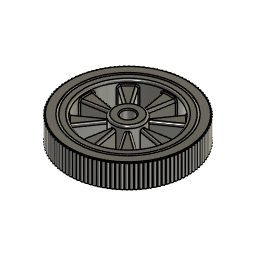
Reifen_Grip_V7 (Autodesk Fusion 360 design; units mm, degrees)
part number: 2025-05-07-17-34-55-146
Autodesk Fusion 360 part; units mm, degrees
note: some values were not read from the file. Chosen so that the rebuilt part matches the saved one: that a step has no effect.
sketch "Skizze1" plane through (0, 0, 0) normal (0, 0, 1) x (1, 0, 0)
  circle A0 centre (0, 0) radius 17
  circle A1 centre (0, 0) radius 14
  circle A2 centre (0, 0) radius 5
  circle A3 centre (0, 0) radius 2.1
  line L0 (-13.8696, -1.9063) -> (-7.5114, -0.5773)
  line L1 (16.2005, -5.1522) -> (10.483, -4.0435)
  line L2 (10.483, -4.0435) -> (16.2005, -5.1522)
  line L3 (0.8682, 4.924) -> (2.4311, 13.7873)
  line L4 (-0.8682, 4.924) -> (-2.4311, 13.7873)
  line L5 (-2.952, 16.7417) -> (-1.918, 10.8776)
  line L6 (-1.918, 10.8776) -> (-2.952, 16.7417)
  line L7 (-2.4311, 13.7873) -> (-0.8682, 4.924)
  line L8 (-2.8679, 4.0958) -> (-8.0301, 11.4681)
  line L9 (-4.0958, 2.8679) -> (-11.4681, 8.0301)
  line L10 (-4.924, 0.8682) -> (-13.7873, 2.4311)
  line L11 (-4.924, -0.8682) -> (-13.7873, -2.4311)
  line L12 (4.924, -0.8682) -> (13.7873, -2.4311)
  line L13 (4.924, 0.8682) -> (13.7873, 2.4311)
  line L14 (-0.8682, -4.924) -> (-2.4311, -13.7873)
  line L15 (0.8682, -4.924) -> (2.4311, -13.7873)
  line L16 (-2.8679, -4.0958) -> (-8.0301, -11.4681)
  line L17 (-4.0958, -2.8679) -> (-11.4681, -8.0301)
  line L18 (2.8211, -4.1281) -> (7.8991, -11.5587)
  line L19 (4.0629, -2.9143) -> (11.3761, -8.16)
  line L20 (4.0958, 2.8679) -> (11.4681, 8.0301)
  line L21 (2.8679, 4.0958) -> (8.0301, 11.4681)
  dimension "d1" = 34
  dimension "d2" = 28
  dimension "d3" = 10
  dimension "d4" = 4.2
  constraint coincident A0.centre A1.centre
  constraint concentric A0 A2
  constraint concentric A2 A3
  constraint coincident A1 L0.start
  constraint coincident A0 L1.start
  constraint parallel L4 L6
  constraint coincident A2 L4.start
  constraint coincident A2 L3.start
  constraint coincident A1 L4.end
  constraint coincident A0 L5.start
  constraint collinear L4 L5
  constraint collinear L6 L7
  constraint coincident A1 L3.end
  constraint coincident A2 L8.start
  constraint coincident A2 L9.start
  constraint coincident A1 L8.end
  constraint coincident A1 L9.end
  constraint coincident A2 L10.start
  constraint coincident A2 L11.start
  constraint coincident A1 L10.end
  constraint coincident A1 L11.end
  constraint coincident A2 L12.start
  constraint coincident A2 L13.start
  constraint coincident A1 L12.end
  constraint coincident A1 L13.end
  constraint coincident A1 L14.end
  constraint coincident A2 L14.start
  constraint coincident A1 L15.end
  constraint coincident A2 L15.start
  constraint coincident A2 L16.start
  constraint coincident A2 L17.start
  constraint coincident A1 L17.end
  constraint coincident A1 L16.end
  constraint coincident A2 L18.start
  constraint coincident A2 L19.start
  constraint coincident A1 L18.end
  constraint coincident A1 L19.end
  constraint coincident A2 L20.start
  constraint coincident A2 L21.start
  constraint coincident A1 L21.end
  constraint coincident A1 L20.end
  measures "d1" diameter of A0
  measures "d2" diameter of A1
  measures "d3" diameter of A2
  measures "d4" diameter of A3
extrude "Extrusion3" add sketch "Skizze1" along normal blind 4 contours A2 makes body 1
extrude "Extrusion4" add sketch "Skizze1" along normal blind 2.5 contours A1 A2 L3 L4 L5 L6 L7 | A1 A2 L8 L9 | A1 A2 L18 L19 | A1 A2 L12 L13 | A1 A2 L20 L21 | A1 A2 L10 L11 | A1 A2 L14 L15 | A1 A2 L16 L17 bodies 1
extrude "Extrusion5" add sketch "Skizze1" along normal blind 4 contours A0 A1 L1 L2 L5 L6 | A0 A1 L1 L2 L5 L6 bodies 1
fillet "Abrundung1" radius 0.7 19 edges at (1.6497, 9.3557, 2.5) (-1.6497, 9.3557, 2.5) (-5.449, 7.7819, 2.5) (-7.7819, 5.449, 2.5) (-9.3557, 1.6497, 2.5) (-9.3557, -1.6497, 2.5) (-7.7819, -5.449, 2.5) (-5.449, -7.7819, 2.5) (-1.6497, -9.3557, 2.5) (1.6497, -9.3557, 2.5) (5.3601, -7.8434, 2.5) (7.7195, -5.5371, 2.5) (9.3557, -1.6497, 2.5) (9.3557, 1.6497, 2.5) (7.7819, 5.449, 2.5) (5.449, 7.7819, 2.5) (-4.6616, -1.8081, 4) (-13.0526, 5.0626, 4) (-15.8496, -6.1475, 4) on bodies 1
fillet "Abrundung2" radius 0.35 40 edges at (2.4311, 13.7873, 0.9) (2.2288, 13.8214, 2.2951) (0, 14, 2.5) (-2.2288, 13.8214, 2.2951) (-2.4311, 13.7873, 0.9) (-8.0301, 11.4681, 0.9) (-8.1972, 11.3492, 2.2951) (-9.8995, 9.8995, 2.5) (-11.3492, 8.1972, 2.2951) (-11.4681, 8.0301, 0.9) (11.4681, 8.0301, 0.9) (11.3492, 8.1972, 2.2951) (9.8995, 9.8995, 2.5) (8.1972, 11.3492, 2.2951) (8.0301, 11.4681, 0.9) (-13.7873, 2.4311, 0.9) (-13.8214, 2.2288, 2.2951) (-14, 0, 2.5) (-13.8214, -2.2288, 2.2951) (-13.7873, -2.4311, 0.9) (-11.4681, -8.0301, 0.9) (-11.3492, -8.1972, 2.2951) (-9.8995, -9.8995, 2.5) (-8.1972, -11.3492, 2.2951) (-8.0301, -11.4681, 0.9) (-2.4311, -13.7873, 0.9) (-2.2288, -13.8214, 2.2951) (0, -14, 2.5) (2.2288, -13.8214, 2.2951) (2.4311, -13.7873, 0.9) (13.7873, -2.4311, 0.9) (13.8214, -2.2288, 2.2951) (14, 0, 2.5) (13.8214, 2.2288, 2.2951) (13.7873, 2.4311, 0.9) (7.8991, -11.5587, 0.9) (8.0677, -11.4417, 2.2951) (9.7863, -10.0114, 2.5) (11.2553, -8.3258, 2.2951) (11.3761, -8.16, 0.9) on bodies 1
fillet "Abrundung3" radius 0.3 1 edges at (-1.9579, 0.7594, 4) on bodies 1
ref_plane "Arbeitsebene1" through (0, 0, 0.3) normal (0, 0, 1) x (1, 0, 0)
sketch "Skizze3" plane through (0, 0, 0.3) normal (0, 0, 1) x (1, 0, 0)
extrude "Extrusion8" add 1 faces at (-7.7001, -7.2908, 0) along direction (0, 0, -1) blind 4 on bodies 1 bodies 1
extrude "Extrusion9" [no effect]
extrude "Extrusion10" [no effect]
sketch "Skizze4" plane through (0, 0, 0) normal (0, 0, 1) x (1, 0, 0)
  circle A0 centre (-19.5, 0) radius 0.4
  dimension "d92" = 0.8
  measures "d92" diameter of A0
sketch "Skizze5" plane through (0, 0, 0) normal (0, 0, 1) x (1, 0, 0)
  circle A0 centre (0, 0) radius 19.5
  circle A1 centre (0, 0) radius 17
  dimension "d99" = 39
  dimension "d100" = 34
  constraint coincident A0.centre A1.centre
  constraint concentric A0 A1
  measures "d99" diameter of A0
  measures "d100" diameter of A1
extrude "Extrusion13" add sketch "Skizze5" along normal blind 4 separate body makes body 2
extrude "Extrusion14" add 1 faces at (18.5308, -1.8133, 0) along direction (0, 0, -1) blind 4 on bodies 2 bodies 2
sketch "Skizze6" plane through (0, 0, 0) normal (0, 0, 1) x (1, 0, 0)
  circle A0 centre (19.5, 0) radius 0.4
  dimension "d105" = 0.8
  measures "d105" diameter of A0
extrude "Extrusion15" add sketch "Skizze6" along normal blind 3.8 bodies 2
extrude "Extrusion16" add 1 faces at (19.6277, 0.0822, 0) along direction (0, 0, -1) blind 3.8 on bodies 2 bodies 2
pattern_circular "C-Anordnung3" count 110 over 360 about axis through (0, 0, -4) along (0, 0, 1) of "Extrusion15", "Extrusion16"
extrude "Extrusion6" [suppressed]
fillet "Abrundung4" [suppressed]
pattern_circular "C-Anordnung1" [suppressed]
extrude "Extrusion7" [suppressed]
named bodies: "Felge"
